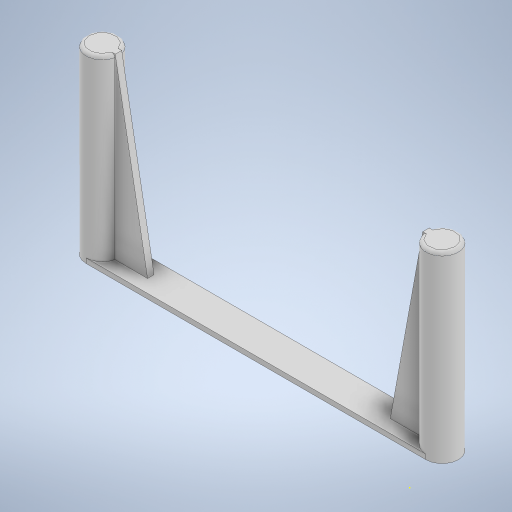
# Autodesk Inventor part: Soporte Platos
Saved by Autodesk Inventor 2024 (Build 280153000, 153)
## iProperties
Created: 2025-02-22
Part Number: Soporte Platos
Material: Genérico
Document SubType Name: Modeling
Designer: sergi
Density: 1 g/cm^3
Appearance: Valor por defecto
Author: sergi
Autodesk Inventor part; units mm, degrees
ref_plane "YZ Plane" through (0, 0, 0) normal (1, 0, 0) x (0, 1, 0)
ref_plane "XZ Plane" through (0, 0, 0) normal (0, 1, 0) x (-1, 0, 0)
ref_plane "XY Plane" through (0, 0, 0) normal (0, 0, 1) x (1, 0, 0)
sketch "Boceto1" plane through (0, 0, 0) normal (0, 1, 0) x (-1, 0, 0)
  line L0 (0, 0) -> (230, 0)
  line L1 (230, 0) -> (230, -760)
  line L2 (230, -760) -> (0, -760)
  line L3 (0, -760) -> (0, 0)
  dimension "d0" = 760
  dimension "d1" = 230
  constraints: 8 end point, 2 parallel, 1 horizontal, 1 perpendicular
  measures "d0" distance of L0.end L1.end
  measures "d1" distance of L1.end L2.end
extrude "Extrusión1" add sketch "Boceto1" along normal blind 3
sketch "Boceto2" plane through (0, 3, 0) normal (0, 1, 0) x (1, 0, 0)
  point P0 (0, 0)
sketch "Boceto3" plane through (0, 3, 0) normal (0, 1, 0) x (1, 0, 0)
  line L0 (0, 760) -> (-230, 760) projected
  line L1 (-230, 760) -> (-230, 0) projected
  line L2 (-230, 0) -> (0, 0) projected
  line L3 (0, 0) -> (0, 760) projected
  line L4 (-20, 20) -> (-210, 20)
  line L5 (-210, 20) -> (-210, 740)
  line L6 (-210, 740) -> (-20, 740)
  line L7 (-20, 740) -> (-20, 20)
  line L8 (0, 20) -> (-230, 20)
  line L9 (-230, 20) -> (-230, 40)
  line L10 (-230, 40) -> (0, 40)
  line L11 (0, 40) -> (0, 20)
  dimension "d4" = 20
  dimension "d5" = 20
  constraints: 16 end point, 3 point on line, 2 parallel, 1 horizontal, 1 perpendicular, 3 other
  measures "d4" distance between parallel lines of L2 L4
  measures "d5" distance of L8.end L9.end
extrude "Extrusión2" add sketch "Boceto3" along normal blind 3 contours L3 L8 L7 L10 | L10 L5 L8 L1 | L7 L4 L5 L10
sketch "Boceto4" plane through (0, 6, 0) normal (0, 1, 0) x (1, 0, 0)
  line L0 (-230, 40) -> (-230, 20) projected
  line L1 (-230, 20) -> (0, 20) projected
  line L2 (0, 20) -> (0, 40) projected
  line L3 (0, 40) -> (-230, 40) projected
  circle A0 centre (-10, 30) radius 10
  line L4 (0, 40) -> (-230, 40) projected
  line L5 (0, 20) -> (0, 40) projected
  circle A1 centre (-220, 30) radius 10
  line L6 (-230, 40) -> (-230, 20) projected
  point P0 (0, 0)
  dimension "d8" = 20
  dimension "d9" = 20
  constraints: 4 tangent, 2 centre point
  measures "d8" diameter of A0
  measures "d9" diameter of A1
extrude "Extrusión3" add sketch "Boceto4" along normal blind 110 contours A1 | A0
sketch "Boceto5" plane through (0, 6, 0) normal (0, 1, 0) x (1, 0, 0)
  circle A0 centre (-220, 30) radius 10 projected
  arc A1 (-10, 40) -> (-10, 20) centre (-10, 30) ccw projected
  line L0 (-10, 40) -> (-220, 40) projected
  arc A2 (-220, 20) -> (-220, 40) centre (-220, 30) ccw projected
  line L1 (-220, 20) -> (-10, 20) projected
  arc A3 (-220, 20) -> (-220, 40) centre (-220, 30) ccw projected
  line L2 (-210, 30) -> (-190, 30)
  line L3 (-190, 30) -> (-190, 32)
  line L4 (-190, 32) -> (-190, 28)
  line L5 (-190, 28) -> (-210.202, 28)
  line L6 (-190, 32) -> (-210.202, 32)
  point P0 (0, 0)
  dimension "d12" = 20
  dimension "d13" = 2
  dimension "d14" = 4
  constraints: 10 end point, 4 point on circle, 3 horizontal, 1 perpendicular, 1 point on line
  measures "d12" distance of L2.start L2.end
  measures "d13" distance of L2.end L3.end
  measures "d14" distance of L3.end L4.end
extrude "Extrusión4" add sketch "Boceto5" along normal up to surface (110 mm away) contours L2 L4 L5 A0 | A0 L6 L3 L2
chamfer "Chaflán2" distance 110 distance2 20 1 edges at (-190, 116, -30) measured on face at (-190, 115.5, -30)
ref_plane "Plano de trabajo1" through (-115, 0, 0) normal (1, 0, 0) x (0, 0, -1)
mirror "Simetría1" about plane through (-115, 0, 0) normal (1, 0, 0) of "Extrusión4", "Chaflán2"
fillet "Empalme1" radius 2 2 edges at (0, 116, -30) (-230, 116, -30)
sketch "Boceto6" plane through (0, 0, 0) normal (0, -1, 0) x (1, 0, 0)
  line L0 (-210, -28) -> (-212.254, -28) projected
  line L1 (-210, -32) -> (-210, -28) projected
  line L2 (-212.254, -32) -> (-210, -32) projected
  arc A0 (-212.254, -28) -> (-212.254, -32) centre (-220, -30) ccw projected
  line L3 (-17.746, -32) -> (-20, -32) projected
  line L4 (-20, -28) -> (-20, -32) projected
  line L5 (-20, -28) -> (-17.746, -28) projected
  arc A1 (-17.746, -32) -> (-17.746, -28) centre (-10, -30) ccw projected
  point P0 (0, 0)
hole "Agujero1" at (-220, 0, -30) at (-10, 0, -30) direction (0, 1, 0) diameter 4 depth 20 tip angle 118
sketch "Boceto7" plane through (0, 6, 0) normal (0, 1, 0) x (1, 0, 0)
  arc A0 (-10, 20) -> (0, 30) centre (-10, 30) ccw projected
  line L0 (-10, 20) -> (0, 20) projected
  line L1 (0, 20) -> (0, 30) projected
  arc A1 (0, 30) -> (-10, 40) centre (-10, 30) ccw projected
  line L2 (0, 30) -> (0, 40) projected
  line L3 (0, 40) -> (-10, 40) projected
  arc A2 (-220, 40) -> (-230, 30) centre (-220, 30) ccw projected
  line L4 (-220, 40) -> (-230, 40) projected
  line L5 (-230, 40) -> (-230, 30) projected
  arc A3 (-230, 30) -> (-220, 20) centre (-220, 30) ccw projected
  line L6 (-230, 30) -> (-230, 20) projected
  line L7 (-230, 20) -> (-220, 20) projected
  point P0 (0, 0)
extrude "Extrusión5" cut sketch "Boceto7" against normal blind 3
ref_plane "Plano de trabajo2" through (0, 3, 0) normal (0, 1, 0) x (1, 0, 0)
split "Dividir1" plane through (0, 3, 0) removes the side toward (0, -1, 0)
